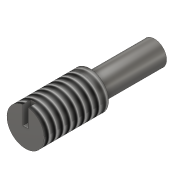
# Autodesk Inventor part: VS-010 (SET SCREW)
Saved by Autodesk Inventor 2017 (Build 210142000, 142)
## iProperties
Created: 2016-12-07
Part Number: VS-010 (SET SCREW)
Material: Steel, Carbon
Document SubType Name: Modeling
Designer: OCCC
Density: 7.85 g/cm^3
Appearance: Semi-Polished
Author: OCCC
Autodesk Inventor part; units mm, degrees
ref_plane "YZ Plane" through (0, 0, 0) normal (1, 0, 0) x (0, 1, 0)
ref_plane "XZ Plane" through (0, 0, 0) normal (0, 1, 0) x (-1, 0, 0)
ref_plane "XY Plane" through (0, 0, 0) normal (0, 0, 1) x (1, 0, 0)
sketch "Sketch1" plane through (0, 0, 0) normal (0, 0, 1) x (1, 0, 0)
  circle A0 centre (0, 0) radius 2.7432
  dimension "d0" = 5.4864
  constraints: 1 centre point, 1 coincident
  measures "d0" diameter of A0
extrude "Extrusion1" add sketch "Sketch1" against normal blind 9.525
sketch "Sketch2" plane through (0, 0, -9.525) normal (0, 0, -1) x (-1, 0, 0)
  circle A0 centre (0, 0) radius 1.7907
  dimension "d3" = 3.5814
  constraints: 1 centre point, 1 coincident
  measures "d3" diameter of A0
extrude "Extrusion2" add sketch "Sketch2" along normal blind 9.525
thread "Thread1" size "12-24 UNC" class "2A" standard "ANSI Unified Screw Threads" length 9.525 offset 1.1906
thread "Thread2" size "12-24 UNC" class "2A" standard "ANSI Unified Screw Threads" full length
sketch "Sketch3" plane through (0, 0, 0) normal (0, 0, 1) x (1, 0, 0)
  line L0 (0, 0) -> (0, 3.3215) construction
  line L1 (-0.3969, 2.772) -> (0.3969, 2.772)
  line L2 (0.3969, 2.772) -> (0.3969, 0)
  line L3 (0.3969, 0) -> (-0.3969, 0)
  line L4 (-0.3969, 0) -> (-0.3969, 2.772)
  dimension "d10" = 0.3969
  dimension "d11" = 0.7937
  constraints: 10 end point, 2 parallel, 1 horizontal, 1 midpoint, 1 perpendicular, 1 vertical
  measures "d10" distance between parallel lines of L2 L0
  measures "d11" distance between parallel lines of L2 L4
extrude "Extrusion3" cut sketch "Sketch3" against normal blind 1.1906
body "Solid1"
